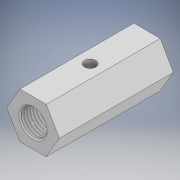
# Autodesk Inventor part: Luftregler1
Saved by Autodesk Inventor 2021 (Build 250183000, 183)
## iProperties
Created: 2021-10-22
Part Number: Luftregler1
Material: Generisch
Document SubType Name: Modeling
Designer: lukas
Density: 1 g/cm^3
Appearance: Vorgabe
Author: lukas
Autodesk Inventor part; units mm, degrees
ref_plane "YZ Plane" through (0, 0, 0) normal (1, 0, 0) x (0, 1, 0)
ref_plane "XZ Plane" through (0, 0, 0) normal (0, 1, 0) x (-1, 0, 0)
ref_plane "XY Plane" through (0, 0, 0) normal (0, 0, 1) x (1, 0, 0)
sketch "Skizze1" plane through (0, 0, 0) normal (0, 0, 1) x (1, 0, 0)
  line L0 (-16.1655, 0) -> (16.1655, 0) projected
  line L1 (0, -14.0455) -> (0, 14.0455) projected
  line L2 (-5.7168, 10.0325) -> (5.83, 9.9672)
  line L3 (5.83, 9.9672) -> (11.5468, -0.0653)
  line L4 (11.5468, -0.0653) -> (5.7168, -10.0325)
  line L5 (5.7168, -10.0325) -> (-5.83, -9.9672)
  line L6 (-5.83, -9.9672) -> (-11.5468, 0.0653)
  line L7 (-11.5468, 0.0653) -> (-5.7168, 10.0325)
  point P0 (0, 0)
  point P1 (0, 0)
  dimension "d0" = 20
  constraints: 12 end point, 1 coincident, 13 other
  measures "d0" distance between parallel lines of L5 L2
extrude "Extrusion1" add sketch "Skizze1" along normal blind 50
sketch "Skizze2" plane through (-5.7168, 10.0325, 50) normal (0.0056567, 0.999984, 0) x (0.999984, -0.0056567, 0)
  line L0 (11.547, 0) -> (0, 0) projected
  circle A0 centre (5.7735, 25) radius 2.5
  point P0 (5.7735, 50)
  dimension "d3" = 25
  dimension "d4" = 5
  constraints: 1 centre point, 1 coincident
  measures "d3" distance from line of point (5.774, 25) L0
  measures "d4" diameter of A0
extrude "Extrusion2" cut sketch "Skizze2" against normal blind 10
sketch "Skizze3" plane through (0, 0, 0) normal (0, 0, -1) x (-1, 0, 0)
  point P0 (0, 0)
hole "Bohrung1" at (0, 0, 0) direction (0, 0, 1) diameter 11.445 depth 40 thread size "G13.157x1.337" designation "G 1/4" standard "ISO Pipe Threads"
sketch "Skizze4" plane through (0, 0, 50) normal (0, 0, 1) x (1, 0, 0)
  point P0 (0, 0)
hole "Bohrung2" at (0, 0, 50) direction (0, 0, -1) diameter 11.445 depth 40 thread size "G13.157x1.337" designation "G 1/4" standard "ISO Pipe Threads"
chamfer "Fase1" distance 0.5 angle 45 1 edges at (0, -5.7225, 0)
chamfer "Fase2" distance 0.5 angle 45 1 edges at (0, 5.7225, 50)
sketch "Skizze5" plane through (0, 0, 50) normal (0, 0, 1) x (1, 0, 0)
  point P0 (0, 0)
